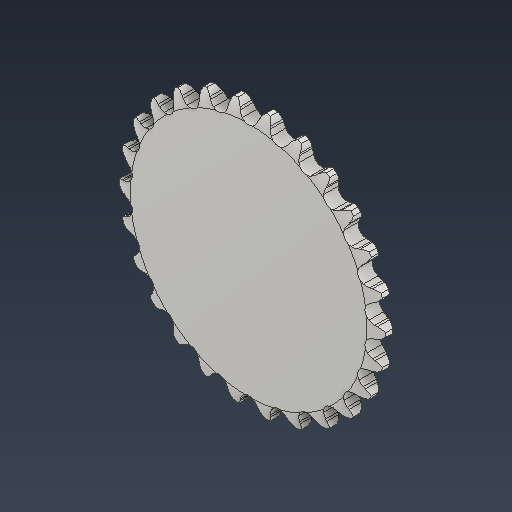
# Autodesk Inventor part: Звездочка роликовой цепи1
Saved by Autodesk Inventor 2025 (Build 290162000, 162)
## iProperties
Created: 2025-03-14
Part Number: Звездочка роликовой цепи1
Material: Steel
Document SubType Name: Modeling
Designer: GameHD
Density: 1 g/cm^3
Appearance: Steel
CustomPartVersion: 1
Author: GameHD
Autodesk Inventor part; units mm, degrees
ref_plane "YZ Plane" through (0, 0, 0) normal (1, 0, 0) x (0, 1, 0)
ref_plane "XZ Plane" through (0, 0, 0) normal (0, 1, 0) x (-1, 0, 0)
sketch "Теоретический профиль зуба" plane through (0, 0, 0) normal (0, 0, 1) x (1, 0, 0)
  circle A0 centre (0, 0) radius 26.3405 construction
  line L0 (0, 0) -> (0, 26.3405) construction
  line L1 (0, 0) -> (6.3037, 25.5751) construction
  circle A1 centre (0, 0) radius 28.0535
  arc A2 (-1.3501, 25.3118) -> (1.3501, 25.3118) centre (0, 26.3405) ccw
  line L2 (0, 26.3405) -> (6.3037, 25.5751) construction
  line L3 (0, 26.3405) -> (2.1011, 27.9416) construction
  line L4 (2.1011, 27.9416) -> (-1.937, 26.3541) construction
  arc A3 (2.9478, 27.8982) -> (2.0977, 26.7628) centre (4.5891, 25.7833) ccw
  arc A4 (-2.0977, 26.7628) -> (-2.9478, 27.8982) centre (-4.5891, 25.7833) ccw
  line L5 (-4.5891, 25.7833) -> (-2.0977, 26.7628) construction
  arc A5 (-1.937, 26.3541) -> (-1.3501, 25.3118) centre (2.1011, 27.9416) ccw
  line L6 (-1.937, 26.3541) -> (-2.0977, 26.7628)
  arc A6 (1.3501, 25.3118) -> (1.937, 26.3541) centre (-2.1011, 27.9416) ccw
  line L7 (2.0977, 26.7628) -> (1.937, 26.3541)
  line L8 (0, 0) -> (3.3815, 27.8489) construction
  point P0 (3.1519, 25.9578)
  dimension "d0" = 52.6811
  dimension "d2" = 13.846
  dimension "d3" = 1.6974
  dimension "d10" = 127.308
  dimension "d11" = 15.846
  dimension "d12" = 2.6416
  dimension "d13" = 4.339
  dimension "d14" = 4.6228
  dimension "d23" = 1.905
  constraints: 18 end point, 15 point on circle, 7 centre point, 3 coincident, 3 point on line, 3 symmetric about line, 3 tangent, 1 equal radius, 1 midpoint, 1 parallel, 1 vertical, 1 other
  measures "d0" diameter of A0
  measures "d2" angle of L1 L0
  measures "d3" radius of A2
  measures "d10" angle of L3 L0
  measures "d11" angle of L4 L3
  measures "d12" distance of L2.start L3.end
  measures "d13" distance of L3.end L4.end
  measures "d14" distance of A3.centre L0.end
  measures "d23" distance from line of L8.end L2
sketch "Профиль зуба" plane through (0, 0, 0) normal (0, 0, 1) x (1, 0, 0)
  arc A0 (-1.5767, 25.7121) -> (1.5767, 25.7121) centre (0, 26.3405) ccw
  arc A1 (2.7595, 27.9174) -> (1.5767, 25.7121) centre (11.883, 21.6043) ccw
  arc A2 (-1.5767, 25.7121) -> (-2.7595, 27.9174) centre (-11.883, 21.6043) ccw
  line L0 (0, 0) -> (0, 26.3405) construction
  line L1 (0, 26.3405) -> (1.5767, 25.7121) construction
  line L2 (0, 26.3405) -> (-1.5767, 25.7121) construction
  circle A3 centre (0, 0) radius 28.0535 projected
  dimension "d44" = 136.538
  dimension "d45" = 11.0947
  dimension "d46" = 1.6974
  constraints: 9 point on circle, 6 end point, 3 centre point, 2 tangent, 1 coincident, 1 equal radius, 1 vertical, 1 other
  measures "d44" angle of L2 L1
  measures "d45" radius of A1
  measures "d46" radius of A0
sketch "Профиль сечения" plane through (0, 0, 0) normal (1, 0, 0) x (0, 1, 0)
  line L0 (28.0535, 0) -> (-28.0535, 0) projected
  line L1 (22.3385, 1.5526) -> (-22.3385, 1.5526)
  line L2 (-22.3385, 1.5526) -> (-22.3385, -1.5526)
  line L3 (-22.3385, -1.5526) -> (22.3385, -1.5526)
  line L4 (22.3385, -1.5526) -> (22.3385, 1.5526)
  line L5 (22.3385, 1.5526) -> (28.0535, 1.5526) construction
  line L6 (28.0535, 1.5526) -> (28.0535, -1.5526) construction
  line L7 (28.0535, -1.5526) -> (22.3385, -1.5526) construction
  line L8 (22.3385, -1.5526) -> (22.3385, 1.5526)
  arc A0 (28.0535, 0.7588) -> (24.8777, 1.5526) centre (24.8777, -5.1975) ccw
  arc A1 (24.8777, -1.5526) -> (28.0535, -0.7588) centre (24.8777, 5.1975) ccw
  line L9 (24.8777, 1.5526) -> (0, 1.5526)
  line L10 (0, 1.5526) -> (0, -1.5526)
  line L11 (0, -1.5526) -> (24.8777, -1.5526)
  line L12 (0, 1.5526) -> (0, -1.5526)
  line L13 (28.0535, 0.7588) -> (28.0535, -0.7588)
  point P0 (0, 0)
  point P1 (0, 0)
  dimension "d30" = 3.1052
  dimension "d31" = 44.677
  dimension "d32" = 3.1052
  dimension "d33" = 0.7937
  dimension "d34" = 6.75
  dimension "d43" = 1.5526
  constraints: 26 end point, 7 midpoint, 5 perpendicular, 4 parallel, 4 point on circle, 3 point on line, 3 symmetric about line, 2 centre point, 2 horizontal, 2 tangent, 1 collinear, 1 other
  measures "d30" distance between parallel lines of L7 L5
  measures "d31" distance between parallel lines of L2 L4
  measures "d32" distance between parallel lines of L3 L1
  measures "d33" distance from line of L13.start L5
  measures "d34" radius of A0
  measures "d43" distance between parallel lines of L3 L0
revolve "Диск" add sketch "Профиль сечения" angle 360 about axis through (0, 0, 1.5526) along (0, 0, -1) contours L10 L3 L2 L0 | L0 L2 L1 L10
revolve "Ветвь" add sketch "Профиль сечения" angle 360 about axis through (0, 0, 1.5526) along (0, 0, -1) contours L13 A1 L11 L4 L0 | L0 L4 L9 A0 L13 | L4 L3 L10 L0 | L0 L10 L1 L4
fillet "Fillet2" [suppressed]
pattern_of_one "Массив ветвей"
extrude "Теоретический зуб" cut sketch "Теоретический профиль зуба" along normal through all both and the other way through all contours A3 L7 A6 A2 A5 L6 A4 A1 picked at (0.3281, 26.4392)
extrude "Зуб" [suppressed]
pattern_circular "Форма зуба" count 26 over 360 about axis through (0, 0, -10) along (0, 0, 1) of "Теоретический зуб"
ref_plane "Плоскость синхронизации" through (0, 26.3405, 0) normal (1, 0, 0) x (0, 1, 0)
equation "\"d3\" = 0.5 * da_Dr + da_SC"
equation "\"d12\" = 0.8 * da_Dr"
equation "\"d13\" = 1.3 * da_Dr + da_SC"
equation "\"d14\" = 1.4 * da_Dr"
equation "\"d23\" = da_Ha"
equation "\"d44\" = da_Alfa"
equation "\"d45\" = da_Re"
equation "\"d46\" = da_Ri"
equation "\"d30\" = da_Bf"
equation "\"d31\" = da_Ds"
equation "\"d32\" = da_Bs"
equation "\"d33\" = da_Ba"
equation "\"d34\" = da_Rx"
equation "\"d51\" = da_Ra"
equation "\"d40\" = da_pt"
equation "\"form_type\" = 0"
equation "\"da_p\" = 6.35"
equation "\"da_Dr\" = 3.302"
equation "\"da_SC\" = 0.04636"
equation "\"da_Ha\" = 1.905"
equation "\"da_pt\" = 6.4008"
equation "\"da_Bf\" = 3.10515"
equation "\"da_Ba\" = 0.79375"
equation "\"da_Rx\" = 6.75005"
equation "\"da_Ra\" = 0.254"
equation "\"da_Bs\" = 3.10515"
equation "\"da_Ds\" = 44.67696"
equation "\"da_Re\" = 11.09472"
equation "\"da_Ri\" = 1.69736"
equation "\"da_Alfa\" = 136.538deg"
body "Solid1"
